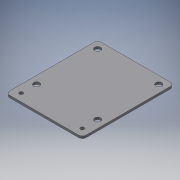
# Autodesk Inventor part: LRFマウント
Saved by Autodesk Inventor 2017 (Build 210142000, 142)
## iProperties
Part Number: LRFマウント
Material: 一般
Document SubType Name: Modeling
Designer: highs
Density: 1 g/cm^3
Appearance: 既定
Author: highs
Autodesk Inventor part; units mm, degrees
ref_plane "YZ Plane" through (0, 0, 0) normal (1, 0, 0) x (0, 1, 0)
ref_plane "XZ Plane" through (0, 0, 0) normal (0, 1, 0) x (-1, 0, 0)
ref_plane "XY Plane" through (0, 0, 0) normal (0, 0, 1) x (1, 0, 0)
sketch "スケッチ1" plane through (0, 0, 0) normal (0, 0, 1) x (1, 0, 0)
  line L0 (0, 0) -> (100, 0)
  line L1 (100, 0) -> (100, 120)
  line L2 (100, 120) -> (0, 120)
  line L3 (0, 120) -> (0, 0)
  line L4 (0, 10) -> (100, 10) construction
  circle A0 centre (10, 10) radius 2.5
  circle A1 centre (90, 10) radius 2.5
  circle A2 centre (10, 110) radius 4
  circle A3 centre (10, 30) radius 4
  circle A4 centre (90, 110) radius 4
  circle A5 centre (90, 30) radius 4
  line L5 (10, 110) -> (10, 30) construction
  line L6 (10, 30) -> (90, 30) construction
  line L7 (90, 30) -> (90, 110) construction
  line L8 (90, 110) -> (10, 110) construction
  dimension "d0" = 5
  dimension "d1" = 10
  dimension "d2" = 10
  dimension "d3" = 10
  dimension "d4" = 100
  dimension "d5" = 120
  dimension "d12" = 8
  dimension "d13" = 10
  dimension "d14" = 10
  dimension "d15" = 10
  dimension "d16" = 10
  dimension "d21" = 80
  constraints: 18 end point, 6 centre point, 4 equal radius, 4 perpendicular, 4 point on line, 2 parallel, 1 horizontal
  measures "d0" diameter of A0
  measures "d1" distance from line of L3 A0.centre
  measures "d2" distance between parallel lines of L0 L4
  measures "d3" distance from line of L1 A1.centre
  measures "d4" distance of L0.start L0.end
  measures "d5" distance of L2.end L0.start
  measures "d12" diameter of A2
  measures "d13" distance from line of L3 L5.start
  measures "d14" distance from line of L2 L5.start
  measures "d15" distance from line of L1 L7.end
  measures "d16" distance from line of L2 L7.end
  measures "d21" distance between parallel lines of L6 L8
extrude "押し出し1" add sketch "スケッチ1" along normal blind 3
fillet "フィレット1" radius 5 4 edges at (100, 120, 1.5) (0, 120, 1.5) (100, 0, 1.5) (0, 0, 1.5)
